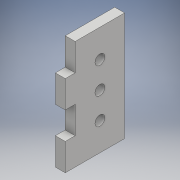
# Autodesk Inventor part: muñeca6
Saved by Autodesk Inventor 2018 (Build 220112000, 112)
## iProperties
Created: 2020-03-11
Part Number: muñeca6
Material: Genérico
Document SubType Name: Modeling
Designer: david
Density: 1 g/cm^3
Appearance: Valor por defecto
Author: david
Autodesk Inventor part; units mm, degrees
ref_plane "YZ Plane" through (0, 0, 0) normal (1, 0, 0) x (0, 1, 0)
ref_plane "XZ Plane" through (0, 0, 0) normal (0, 1, 0) x (-1, 0, 0)
ref_plane "XY Plane" through (0, 0, 0) normal (0, 0, 1) x (1, 0, 0)
sketch "Boceto1" plane through (0, 0, 0) normal (1, 0, 0) x (0, 1, 0)
  line L0 (0, 0) -> (15, 0)
  line L1 (15, 0) -> (15, -33)
  line L2 (15, -33) -> (0, -33)
  circle A0 centre (7.5, -8.5) radius 1.5
  circle A1 centre (7.5, -24.5) radius 1.5
  circle A2 centre (7.5, -16.5) radius 1.5
  line L3 (0, -16.5) -> (-3, -16.5)
  line L4 (-3, -16.5) -> (-3, -8.25)
  line L5 (-3, -24.75) -> (-3, -33)
  line L6 (-3, -33) -> (0, -33)
  line L7 (0, -8.25) -> (-3, -8.25)
  line L8 (-3, -24.75) -> (0, -24.75)
  line L9 (0, 0) -> (0, -8.25)
  line L10 (0, -16.5) -> (0, -24.75)
  dimension "d0" = 33
  dimension "d4" = 3
  dimension "d5" = 3
  dimension "d6" = 3
  dimension "d8" = 8.25
  dimension "d9" = 8.25
  dimension "d10" = 8.25
  dimension "d11" = 8.25
  constraints: 22 end point, 4 perpendicular, 3 centre point, 3 vertical, 2 horizontal, 1 parallel
  measures "d0" distance of L0.start L2.end
  measures "d4" diameter of A0
  measures "d5" diameter of A1
  measures "d6" diameter of A2
  measures "d8" distance of L5.start L5.end
  measures "d9" distance of L3.start L8.end
  measures "d10" distance of L3.end L4.end
  measures "d11" distance of L0.start L7.start
extrude "Extrusión1" add sketch "Boceto1" along normal blind 3
